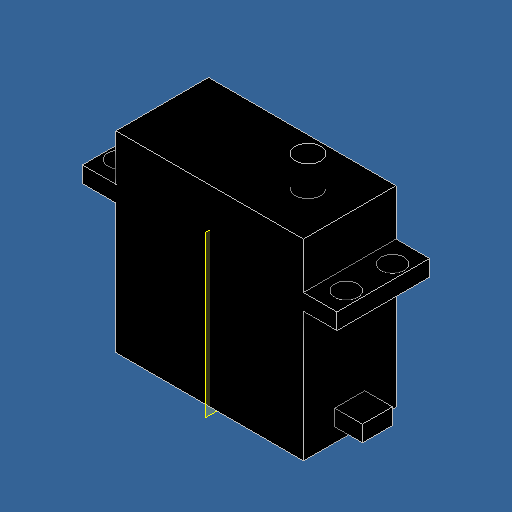
# Autodesk Inventor part: motor_25kg
Saved by Autodesk Inventor 2025 (Build 290162000, 162)
## iProperties
Created: 2024-12-10
Part Number: motor_25kg
Material: Generic
Document SubType Name: Modeling
Designer: Pauline Simonnet
Density: 1 g/cm^3
Appearance: Anodized - Black
Author: Pauline Simonnet
Autodesk Inventor part; units mm, degrees
ref_plane "YZ Plane" through (0, 0, 0) normal (1, 0, 0) x (0, 1, 0)
ref_plane "XZ Plane" through (0, 0, 0) normal (0, 1, 0) x (-1, 0, 0)
ref_plane "XY Plane" through (0, 0, 0) normal (0, 0, 1) x (1, 0, 0)
sketch "Sketch1" plane through (0, 0, 0) normal (0, 1, 0) x (-1, 0, 0)
  line L0 (0, 0) -> (40.5, 0)
  line L1 (40.5, 0) -> (40.5, -20)
  line L2 (40.5, -20) -> (0, -20)
  line L3 (0, -20) -> (0, 0)
  dimension "d0" = 20
  dimension "d1" = 40.5
  constraints: 8 end point, 2 parallel, 1 horizontal, 1 perpendicular
  measures "d0" distance of L0.end L1.end
  measures "d1" distance of L1.end L2.end
extrude "Extrusion1" add sketch "Sketch1" along normal blind 28
sketch "Sketch2" plane through (0, 28, 0) normal (0, 1, 0) x (1, 0, 0)
  line L0 (7.25, 0) -> (-47.75, 0)
  line L1 (-47.75, 0) -> (-47.75, 20)
  line L2 (-47.75, 20) -> (7.25, 20)
  line L3 (7.25, 20) -> (7.25, 0)
  line L4 (0, 20) -> (-40.5, 20) projected
  line L5 (-40.5, 20) -> (-40.5, 0) projected
  line L6 (-40.5, 0) -> (0, 0) projected
  dimension "d4" = 0
  dimension "d5" = 55
  dimension "d6" = 7.25
  dimension "d7" = 0
  constraints: 8 end point, 2 parallel, 1 horizontal, 1 perpendicular
  measures "d4" distance between parallel lines of L4 L2
  measures "d5" distance between parallel lines of L3 L1
  measures "d6" distance between parallel lines of L5 L1
  measures "d7" distance between parallel lines of L0 L6
extrude "Extrusion2" add sketch "Sketch2" along normal blind 3.5
sketch "Sketch3" plane through (0, 31.5, 0) normal (0, 1, 0) x (1, 0, 0)
  circle A0 centre (-44.75, 5) radius 2.5
  circle A1 centre (-44.75, 15) radius 2.5
  line L0 (-47.75, 0) -> (7.25, 0) projected
  line L1 (7.25, 20) -> (-47.75, 20) projected
  line L2 (-47.75, 20) -> (-47.75, 0) projected
  point P0 (0, 0)
  dimension "d10" = 5
  dimension "d11" = 5
  dimension "d12" = 5
  dimension "d14" = 5
  dimension "d15" = 3
  dimension "d16" = 3
  constraints: 2 centre point
  measures "d10" diameter of A1
  measures "d11" diameter of A0
  measures "d12" distance from line of A0.centre L0
  measures "d14" distance from line of L1 A1.centre
  measures "d15" distance from line of A1.centre L2
  measures "d16" distance from line of L2 A0.centre
extrude "Extrusion3" cut sketch "Sketch3" against normal blind 3.5
ref_plane "Work Plane1" through (-20.25, 28, 0) normal (1, 0, 0) x (0, 0, -1)
mirror "Mirror1" about plane through (-20.25, 28, 0) normal (1, 0, 0) of "Extrusion3"
sketch "Sketch4" plane through (0, 31.5, 0) normal (0, 1, 0) x (1, 0, 0)
  line L0 (0, 0) -> (-40.5, 0)
  line L1 (-40.5, 0) -> (-40.5, 20)
  line L2 (-40.5, 20) -> (0, 20)
  line L3 (0, 20) -> (0, 0)
  constraints: 8 end point, 2 parallel, 1 horizontal, 1 perpendicular
extrude "Extrusion4" add sketch "Sketch4" along normal blind 10
sketch "Sketch5" plane through (0, 41.5, 0) normal (0, 1, 0) x (1, 0, 0)
  circle A0 centre (-9, 10) radius 2.75
  line L0 (0, 0) -> (0, 20) projected
  line L1 (-40.5, 0) -> (0, 0) projected
  dimension "d21" = 9
  dimension "d22" = 10
  dimension "d23" = 5.5
  constraints: 1 centre point
  measures "d21" distance from line of A0.centre L0
  measures "d22" distance from line of A0.centre L1
  measures "d23" diameter of A0
extrude "Extrusion5" add sketch "Sketch5" along normal blind 6.5
sketch "Sketch6" plane through (0, 0, 0) normal (1, 0, 0) x (0, 0, -1)
  line L0 (6.75, 3) -> (13.25, 3)
  line L1 (13.25, 3) -> (13.25, 6.5)
  line L2 (13.25, 6.5) -> (6.75, 6.5)
  line L3 (6.75, 6.5) -> (6.75, 3)
  line L4 (0, 0) -> (20, 0) projected
  line L5 (0, 0) -> (0, 28) projected
  dimension "d26" = 3
  dimension "d27" = 6.5
  dimension "d28" = 3.5
  dimension "d29" = 6.75
  constraints: 8 end point, 2 parallel, 1 horizontal, 1 perpendicular
  measures "d26" distance between parallel lines of L0 L4
  measures "d27" distance between parallel lines of L1 L3
  measures "d28" distance of L2.end L0.start
  measures "d29" distance between parallel lines of L3 L5
extrude "Extrusion6" add sketch "Sketch6" along normal blind 6
body "Solid1"
